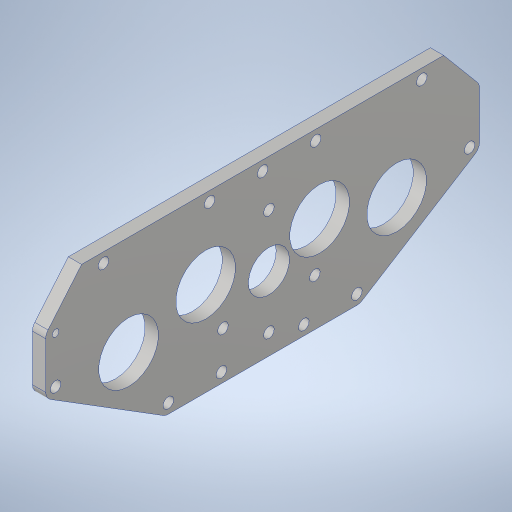
# Autodesk Inventor part: EL2-GB-001
Saved by Autodesk Inventor 2023.4 (Build 274418000, 418)
## iProperties
Created: 2025-01-17
Part Number: EL2-GB-001
Material: Aluminum 6061
Document SubType Name: Modeling
Designer: mavericks
Density: 2.7 g/cm^3
Appearance: Aluminum - Flat
Author: mavericks
Autodesk Inventor part; units mm, degrees
ref_plane "YZ Plane" through (0, 0, 0) normal (1, 0, 0) x (0, 1, 0)
ref_plane "XZ Plane" through (0, 0, 0) normal (0, 1, 0) x (-1, 0, 0)
ref_plane "XY Plane" through (0, 0, 0) normal (0, 0, 1) x (1, 0, 0)
sketch "Sketch1" plane through (0, 0, 0) normal (1, 0, 0) x (0, 1, 0)
  line L0 (-1.5875, -355.6) -> (1.5875, -355.6) construction
  line L1 (1.5875, -355.6) -> (1.5875, 355.6) construction
  line L2 (1.5875, 355.6) -> (-1.5875, 355.6) construction
  line L3 (-1.5875, 355.6) -> (-1.5875, -355.6) construction
  line L4 (-1.5875, -355.6) -> (1.5875, 355.6) construction
  line L5 (1.5875, -355.6) -> (-1.5875, 355.6) construction
  line L6 (52.3875, 152.4) -> (1.5875, 152.4) construction
  line L7 (1.5875, 152.4) -> (1.5875, 127) construction
  line L8 (1.5875, 127) -> (52.3875, 127) construction
  line L9 (52.3875, 127) -> (52.3875, 152.4) construction
  line L10 (52.3875, 152.4) -> (1.5875, 127) construction
  line L11 (1.5875, 152.4) -> (52.3875, 127) construction
  line L12 (77.7875, 177.8) -> (1.5875, 177.8) construction
  line L13 (1.5875, 177.8) -> (1.5875, 152.4) construction
  line L14 (1.5875, 152.4) -> (77.7875, 152.4) construction
  line L15 (77.7875, 152.4) -> (77.7875, 177.8) construction
  line L16 (77.7875, 177.8) -> (1.5875, 152.4) construction
  line L17 (1.5875, 177.8) -> (77.7875, 152.4) construction
  line L18 (900.1125, 152.4) -> (87.3125, 152.4) construction
  line L19 (87.3125, 152.4) -> (87.3125, 177.8) construction
  line L20 (87.3125, 177.8) -> (900.1125, 177.8) construction
  line L21 (900.1125, 177.8) -> (900.1125, 152.4) construction
  line L22 (900.1125, 152.4) -> (87.3125, 177.8) construction
  line L23 (87.3125, 152.4) -> (900.1125, 177.8) construction
  line L24 (87.3125, 177.8) -> (77.7875, 177.8) construction
  line L25 (77.7875, 177.8) -> (77.7875, -177.8) construction
  line L26 (77.7875, -177.8) -> (87.3125, -177.8) construction
  line L27 (87.3125, -177.8) -> (87.3125, 177.8) construction
  line L28 (87.3125, 177.8) -> (77.7875, -177.8) construction
  line L29 (77.7875, 177.8) -> (87.3125, -177.8) construction
  line L30 (82.55, 0) -> (-1.5875, 0) construction
  line L31 (1.5875, -355.6) -> (-1.5875, -355.6) construction
  line L32 (52.3875, -152.4) -> (1.5875, -152.4) construction
  line L33 (1.5875, -152.4) -> (1.5875, -127) construction
  line L34 (1.5875, -127) -> (52.3875, -127) construction
  line L35 (52.3875, -127) -> (52.3875, -152.4) construction
  line L36 (52.3875, -152.4) -> (1.5875, -127) construction
  line L37 (1.5875, -152.4) -> (52.3875, -127) construction
  line L38 (77.7875, -177.8) -> (1.5875, -177.8) construction
  line L39 (1.5875, -177.8) -> (1.5875, -152.4) construction
  line L40 (1.5875, -152.4) -> (77.7875, -152.4) construction
  line L41 (77.7875, -152.4) -> (77.7875, -177.8) construction
  line L42 (77.7875, -177.8) -> (1.5875, -152.4) construction
  line L43 (1.5875, -177.8) -> (77.7875, -152.4) construction
  line L44 (900.1125, -152.4) -> (87.3125, -152.4) construction
  line L45 (87.3125, -152.4) -> (87.3125, -177.8) construction
  line L46 (87.3125, -177.8) -> (900.1125, -177.8) construction
  line L47 (900.1125, -177.8) -> (900.1125, -152.4) construction
  line L48 (900.1125, -152.4) -> (87.3125, -177.8) construction
  line L49 (87.3125, -152.4) -> (900.1125, -177.8) construction
  line L50 (87.3125, -177.8) -> (77.7875, -177.8) construction
  circle A0 centre (66.6623, 160.02) radius 10.3124 construction
  circle A1 centre (66.6623, -160.02) radius 10.3124 construction
  line L51 (138.1125, 176.2125) -> (138.1125, 109.4105) construction
  line L52 (138.1125, 109.4105) -> (-27.5223, 109.4105) construction
  point P0 (0, 0)
  point P1 (26.9875, 139.7)
  point P2 (39.6875, 165.1)
  point P3 (1.5875, 165.1)
  point P4 (493.7125, 165.1)
  point P5 (26.9875, -139.7)
  point P6 (39.6875, -165.1)
  point P7 (1.5875, -165.1)
  point P8 (493.7125, -165.1)
  dimension "d0" = 3.175
  dimension "d1" = 711.2
  dimension "d2" = 50.8
  dimension "d3" = 25.4
  dimension "d4" = 139.7
  dimension "d5" = 76.2
  dimension "d6" = 25.4
  dimension "d7" = 812.8
  dimension "d8" = 25.4
  dimension "d9" = 9.525
  dimension "d10" = 355.6
  dimension "d11" = 20.6248
  dimension "d12" = 11.1252
  dimension "d13" = 7.62
  dimension "d23" = 66.802
  dimension "d24" = 50.8
  constraints: 106 end point, 19 symmetric about line, 12 midpoint, 10 parallel, 7 perpendicular, 6 horizontal, 5 point on line, 3 coincident, 2 centre point, 1 horizontal alignment, 1 other
  measures "d0" distance of L2.end L1.end
  measures "d1" distance of L1.end L0.end
  measures "d2" distance of L8.end L7.end
  measures "d3" distance of L7.end L6.end
  measures "d4" vertical distance of L30.end point (26.988, 139.7)
  measures "d5" distance of L14.end L13.end
  measures "d6" distance of L13.end L12.end
  measures "d7" distance of L19.end L20.end
  measures "d8" distance of L18.end L19.end
  measures "d9" distance of L26.end L25.end
  measures "d10" distance of L25.end L24.end
  measures "d11" diameter of A0
  measures "d12" distance from line of L15 A0.centre
  measures "d13" distance from line of L14 A0.centre
  measures "d23" distance of L51.start L51.end
  measures "d24" distance between parallel lines of L27 L51
sketch "Sketch3" plane through (0, 0, 0) normal (1, 0, 0) x (0, 1, 0)
  line L0 (77.7875, -152.4) -> (77.7875, -177.8) construction
  circle A0 centre (66.6623, -160.02) radius 10.3124 construction
  line L1 (1.5875, 355.6) -> (-1.5875, 355.6) construction
  line L2 (1.5875, -355.6) -> (1.5875, 355.6) construction
  line L3 (-1.5875, -355.6) -> (1.5875, 355.6) construction
  line L4 (1.5875, -355.6) -> (-1.5875, 355.6) construction
  line L5 (-1.5875, 355.6) -> (-1.5875, -355.6) construction
  line L6 (87.3125, -177.8) -> (87.3125, 177.8) construction
  line L7 (77.7875, 177.8) -> (77.7875, -177.8) construction
  line L8 (-1.5875, -355.6) -> (1.5875, -355.6) construction
  line L9 (1.5875, -355.6) -> (-1.5875, -355.6) construction
  line L10 (1.5875, 152.4) -> (1.5875, 127) construction
  line L11 (82.55, 0) -> (-1.5875, 0) construction
  line L12 (87.3125, 152.4) -> (87.3125, 177.8) construction
  line L13 (77.7875, -177.8) -> (87.3125, -177.8) construction
  line L14 (1.5875, -127) -> (52.3875, -127) construction
  line L15 (52.3875, 152.4) -> (1.5875, 152.4) construction
  line L16 (52.3875, 152.4) -> (1.5875, 127) construction
  line L17 (1.5875, 127) -> (52.3875, 127) construction
  line L18 (52.3875, 127) -> (52.3875, 152.4) construction
  line L19 (1.5875, 152.4) -> (52.3875, 127) construction
  line L20 (1.5875, 152.4) -> (77.7875, 152.4) construction
  line L21 (1.5875, 177.8) -> (1.5875, 152.4) construction
  line L22 (138.1125, 109.4105) -> (-27.5223, 109.4105) construction
  circle A1 centre (66.6623, 160.02) radius 10.3124 construction
  line L23 (138.1125, 176.2125) -> (138.1125, 109.4105) construction
  line L24 (77.7875, 177.8) -> (1.5875, 152.4) construction
  line L25 (77.7875, 177.8) -> (1.5875, 177.8) construction
  line L26 (77.7875, 152.4) -> (77.7875, 177.8) construction
  line L27 (87.3125, 177.8) -> (77.7875, 177.8) construction
  line L28 (1.5875, 177.8) -> (77.7875, 152.4) construction
  line L29 (900.1125, 152.4) -> (87.3125, 152.4) construction
  line L30 (87.3125, 177.8) -> (900.1125, 177.8) construction
  line L31 (900.1125, 152.4) -> (87.3125, 177.8) construction
  line L32 (87.3125, 152.4) -> (900.1125, 177.8) construction
  line L33 (900.1125, -152.4) -> (87.3125, -177.8) construction
  line L34 (87.3125, -177.8) -> (900.1125, -177.8) construction
  line L35 (900.1125, -152.4) -> (87.3125, -152.4) construction
  line L36 (87.3125, -152.4) -> (900.1125, -177.8) construction
  line L37 (900.1125, 177.8) -> (900.1125, 152.4) construction
  line L38 (900.1125, -177.8) -> (900.1125, -152.4) construction
  line L39 (52.3875, -127) -> (52.3875, -152.4) construction
  line L40 (52.3875, -152.4) -> (1.5875, -127) construction
  line L41 (1.5875, -152.4) -> (1.5875, -127) construction
  line L42 (1.5875, -152.4) -> (52.3875, -127) construction
  line L43 (52.3875, -152.4) -> (1.5875, -152.4) construction
  line L44 (1.5875, -152.4) -> (77.7875, -152.4) construction
  line L45 (1.5875, -177.8) -> (77.7875, -152.4) construction
  line L46 (77.7875, -177.8) -> (1.5875, -177.8) construction
  line L47 (1.5875, -177.8) -> (1.5875, -152.4) construction
  line L48 (77.7875, -177.8) -> (1.5875, -152.4) construction
  line L49 (87.3125, -152.4) -> (87.3125, -177.8) construction
  line L50 (87.3125, -177.8) -> (77.7875, -177.8) construction
  circle A2 centre (39.6875, 64.1731) radius 28.6512 construction
  circle A3 centre (65.0875, 99.0981) radius 10.3124 construction
  line L51 (57.4199, 164.5943) -> (14.0091, 76.8819) construction
  circle A4 centre (39.6875, 64.1731) radius 25.4 construction
  circle A5 centre (49.2125, 27.2829) radius 12.7 construction
  circle A6 centre (49.2125, 27.2829) radius 25.4 construction
  circle A7 centre (39.6875, -3.0046) radius 6.35 construction
  circle A8 centre (39.6875, -3.0046) radius 25.4 construction
  circle A9 centre (39.6875, -3.0046) radius 30.48 construction
  circle A10 centre (65.0875, 99.0981) radius 4.7625 construction
  circle A11 centre (39.6875, 64.1731) radius 14.2875
  circle A12 centre (49.2125, 27.2829) radius 14.2875
  circle A13 centre (9.2075, 45.1231) radius 4.7625 construction
  circle A14 centre (9.2075, 19.7231) radius 4.7625 construction
  line L52 (87.3125, 0) -> (87.3125, 86.6661)
  line L53 (87.3125, 86.6661) -> (68.1488, 102.7464)
  circle A15 centre (42.8625, 99.0981) radius 4.7625 construction
  line L54 (65.0875, 103.8606) -> (42.8625, 103.8606)
  line L55 (38.8212, 101.6179) -> (5.1662, 47.6429)
  line L56 (4.445, 45.1231) -> (4.445, 0)
  arc A16 (68.1488, 102.7464) -> (65.0875, 103.8606) centre (65.0875, 99.0981) ccw
  arc A17 (42.8625, 103.8606) -> (38.8212, 101.6179) centre (42.8625, 99.0981) ccw
  arc A18 (5.1662, 47.6429) -> (4.445, 45.1231) centre (9.2075, 45.1231) ccw
  line L57 (87.3125, 0) -> (87.3125, -86.6661)
  line L58 (87.3125, -86.6661) -> (68.1488, -102.7464)
  line L59 (65.0875, -103.8606) -> (42.8625, -103.8606)
  line L60 (38.8212, -101.6179) -> (5.1662, -47.6429)
  line L61 (4.445, -45.1231) -> (4.445, 0)
  arc A19 (65.0875, -103.8606) -> (68.1488, -102.7464) centre (65.0875, -99.0981) ccw
  arc A20 (38.8212, -101.6179) -> (42.8625, -103.8606) centre (42.8625, -99.0981) ccw
  arc A21 (4.445, -45.1231) -> (5.1662, -47.6429) centre (9.2075, -45.1231) ccw
  circle A22 centre (39.6875, -3.0046) radius 9.8425
  circle A23 centre (39.6875, -64.1731) radius 14.2875
  circle A24 centre (49.2125, -27.2829) radius 14.2875
  point P0 (0, 0)
  point P1 (0, 0)
  point P2 (26.9875, 139.7)
  point P3 (1.5875, 165.1)
  point P4 (39.6875, 165.1)
  point P5 (493.7125, -165.1)
  point P6 (493.7125, 165.1)
  point P7 (26.9875, -139.7)
  point P8 (1.5875, -165.1)
  point P9 (39.6875, -165.1)
  point P10 (65.0875, -3.0046)
  point P11 (52.3875, 18.9924)
  point P12 (26.9875, 18.9924)
  point P13 (14.2875, -3.0046)
  point P14 (26.9875, -25.0017)
  point P15 (52.3875, -25.0017)
  point P16 (82.55, 76.2)
  point P17 (82.55, 25.4)
  point P18 (82.55, 177.8)
  dimension "d30" = 57.3024
  dimension "d36" = 50.8
  dimension "d31" = 12.7
  dimension "d32" = 50.8
  dimension "d33" = 25.4
  dimension "d34" = 50.8
  dimension "d35" = 12.7
  dimension "d37" = 60.96
  dimension "d38" = 38.1
  dimension "d39" = 34.925
  dimension "d40" = 9.525
  dimension "d41" = 28.575
  dimension "d42" = 28.575
  dimension "d45" = 360
  dimension "d47" = 50.8
  dimension "d48" = 25.4
  dimension "d49" = 22.225
  dimension "d50" = 7.62
  dimension "d51" = 25.4
  dimension "d52" = 19.05
  dimension "d55" = 130
  dimension "d66" = 19.685
  dimension "d68" = 28.575
  dimension "d69" = 38.1
  constraints: 22 end point, 21 centre point, 18 point on circle, 15 coincident, 12 symmetric about line, 8 tangent, 3 equal radius, 3 horizontal alignment, 3 vertical alignment, 1 midpoint, 1 parallel, 1 point on line, 1 vertical, 26 other
  measures "d31" distance from line of L7 A3.centre
  measures "d32" diameter of A4
  measures "d33" diameter of A5
  measures "d34" diameter of A6
  measures "d35" diameter of A7
  measures "d37" diameter of A9
  measures "d38" distance from line of L7 point (39.688, 64.173)
  measures "d39" vertical distance of A3.centre point (39.688, 64.173)
  measures "d40" diameter of A10
  measures "d41" diameter of A11
  measures "d42" diameter of A12
  measures "d47" distance of point (82.55, 25.4) point (82.55, 76.2)
  measures "d48" distance of L11.start point (82.55, 25.4)
  measures "d49" distance of A3.centre point (42.863, 99.098)
  measures "d51" distance of point (9.208, 19.723) point (9.207, 45.123)
  measures "d52" vertical distance of point (39.688, 64.173) point (9.207, 45.123)
  measures "d55" angle of L53 L52
  measures "d66" diameter of A22
  measures "d68" distance from line of L7 A12.centre
extrude "Extrusion1" add sketch "Sketch3" along normal blind 6.35
hole "Mount Holes" at (0, 87.3125, -177.8) at (0, 77.7875, -152.4) at (0, 77.7875, -177.8) at (0, 1.5875, 355.6) at (0, -1.5875, 355.6) at (0, 1.5875, 127) at (0, 1.5875, 152.4) at (0, -27.5223, 109.4105) at (0, 0, 0) at (0, 82.55, 0) at (0, 87.3125, 152.4) at (0, 87.3125, 177.8) at (0, 138.1125, 176.2125) at (0, 52.3875, 152.4) at (0, 26.9875, 139.7) at (0, 52.3875, 127) at (0, 1.5875, 165.1) at (0, 39.6875, 165.1) at (0, 77.7875, 152.4) at (0, 66.6623, 160.02) at (0, 493.7125, -165.1) at (0, 493.7125, 165.1) at (0, 26.9875, -139.7) at (0, 66.6623, -160.02) at (0, 1.5875, -165.1) at (0, 39.6875, -165.1) at (0, 52.3875, -25.0017) at (0, 82.55, 76.2) at (0, 82.55, 25.4) at (0, 42.8625, 99.0981) at (0, 9.2075, 45.1231) at (0, 9.2075, 19.7231) direction (1, 0, 0) diameter 5.1054 end through all clearance for "Flat Head Machine Screw (82)" size "#10" standard "Ansi Unified Screw Threads"
hole "Motor Mount" at (0, 77.7875, -177.8) at (0, 65.0875, -3.0046) at (0, 52.3875, 18.9924) at (0, 26.9875, 18.9924) at (0, 14.2875, -3.0046) at (0, 26.9875, -25.0017) direction (1, 0, 0) diameter 5.1054 end through all clearance for "Flat Head Machine Screw (82)" size "#10" standard "Ansi Unified Screw Threads"
mirror "Mirror1" about plane through (0, 0, 0) normal (0, 0, 1) of "Mount Holes"
hole "Hole3" at (0, 65.0875, 99.0981) direction (1, 0, 0) diameter 3.302 end through all thread size "8-32 UNC" class "2B" standard "ANSI Unified Screw Threads"
body "Solid1"
